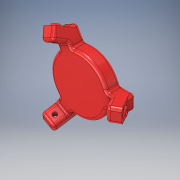
# Autodesk Inventor part: BottomPlatform
Saved by Autodesk Inventor 2019 (Build 230136000, 136)
## iProperties
Created: 2022-07-06
Part Number: BottomPlatform
Material: Generic
Document SubType Name: Modeling
Designer: zreik
Density: 1 g/cm^3
Appearance: Light Red
Author: zreik
Autodesk Inventor part; units mm, degrees
ref_plane "YZ Plane" through (0, 0, 0) normal (1, 0, 0) x (0, 1, 0)
ref_plane "XZ Plane" through (0, 0, 0) normal (0, 1, 0) x (-1, 0, 0)
ref_plane "XY Plane" through (0, 0, 0) normal (0, 0, 1) x (1, 0, 0)
sketch "Sketch1" plane through (0, 0, 0) normal (0, 0, 1) x (1, 0, 0)
  circle A0 centre (0, 0) radius 20
  line L0 (10, -5) -> (30, -5)
  line L1 (30, -5) -> (30, 5)
  line L2 (30, 5) -> (10, 5)
  line L3 (10, 5) -> (10, -5)
  line L4 (10, -5) -> (30, 5) construction
  line L5 (30, -5) -> (10, 5) construction
  point P0 (20, 0)
  dimension "d0" = 40
  dimension "d3" = 10
  dimension "d4" = 20
  dimension "d5" = 0
  constraints: 12 end point, 2 midpoint, 2 parallel, 1 coincident, 1 horizontal, 1 horizontal alignment, 1 perpendicular, 2 other
  measures "d3" distance of L0.end L1.end
  measures "d4" distance of L0.start L0.end
  measures "d5" vertical distance of point (0, 0) point (20, 0)
extrude "Extrusion1" add sketch "Sketch1" along normal mid plane 10 contours A0 L0 L3 L2 | L2 L3 L0 A0
extrude "Extrusion2" add sketch "Sketch1" along normal mid plane 10 contours A0 L0 L3 L2 | A0 L2 L1 L0 picked at (13.3333, 0)
chamfer "Chamfer1" distance 7 angle 30 1 edges at (30, 0, 5) measured on face at (6.3805, 10.8065, 5)
sketch "Sketch2" plane through (23, -5, 5) normal (0.5, 0, 0.8660254) x (0.8660254, 0, -0.5)
  line L0 (8.0829, 0) -> (0, 0)
  line L1 (0, 0) -> (0, 10)
  line L2 (0, 10) -> (8.0829, 10)
  line L3 (8.0829, 10) -> (8.0829, 0)
  line L4 (8.0829, 0) -> (0, 10) construction
  line L5 (0, 0) -> (8.0829, 10) construction
  line L6 (0, 10) -> (0, 0) projected
  line L7 (8.0829, 0) -> (8.0829, 10) projected
  line L8 (8.0829, 10) -> (0, 10) projected
  line L9 (0, 0) -> (8.0829, 0) projected
  point P0 (-17.4186, 5)
  point P1 (4.0415, 5)
  dimension "d11" = 0
  dimension "d12" = 0
  dimension "d13" = 0
  dimension "d14" = 0
  constraints: 12 end point, 2 midpoint, 2 parallel, 1 horizontal, 1 perpendicular
  measures "d11" distance between parallel lines of L1 L6
  measures "d12" distance between parallel lines of L7 L3
  measures "d13" distance between parallel lines of L8 L2
  measures "d14" distance between parallel lines of L9 L0
extrude "Extrusion3" add sketch "Sketch2" along normal blind 10
sketch "Sketch3" plane through (23, -5, 5) normal (-0.8660254, 0, 0.5) x (0.5, 0, 0.8660254)
  circle A0 centre (5, 5) radius 1.5
  line L0 (10, 10) -> (10, 0) projected
  line L1 (0, 10) -> (0, 0) projected
  line L2 (0, 0) -> (10, 0) projected
  line L3 (0, 10) -> (10, 10) projected
  point P0 (-15.8301, 5)
  dimension "d17" = 3
  dimension "d18" = 5
  dimension "d19" = 5
  dimension "d20" = 5
  dimension "d21" = 5
  constraints: 1 centre point
  measures "d17" diameter of A0
  measures "d18" distance from line of L0 A0.centre
  measures "d19" distance from line of L1 A0.centre
  measures "d20" distance from line of L2 A0.centre
  measures "d21" distance from line of L3 A0.centre
extrude "Extrusion8" cut sketch "Sketch3" against normal through all contours A0
sketch "Sketch6" plane through (30, -5, 0.9585) normal (0.8660254, 0, -0.5) x (-0.5, 0, -0.8660254)
  circle A0 centre (-5, 5) radius 3.5
  circle A1 centre (-5, 5) radius 1.5 projected
  point P0 (15.8301, 5)
  dimension "d40" = 7
  constraints: 1 centre point, 1 concentric
  measures "d40" diameter of A0
extrude "Extrusion9" add sketch "Sketch6" along normal blind 1.158
chamfer "Chamfer3" distance 1 angle 45 1 edges at (35.2529, 0, 7.7408)
pattern_circular "Circular Pattern1" count 3 over 360 about axis through (0, 0, 0) along (0, 0, 1) of "Extrusion3", "Extrusion2", "Chamfer1", "Extrusion8", "Chamfer3", "Extrusion9"
fillet "Fillet1" radius 2 9 edges at (30, 0, -5) (-15, 25.9808, -5) (-15, -25.9808, -5) (19.3649, 5, 0) (-5.3523, 19.2705, 0) (19.3649, -5, 0) (-5.3523, -19.2705, 0) (-14.0126, -14.2705, 0) (-14.0126, 14.2705, 0)
fillet "Fillet2" radius 2 3 edges at (-11.5, -19.9186, 5) (23, 0, 5) (-11.5, 19.9186, 5)
fillet "Fillet3" radius 2 3 edges at (-14, 24.2487, 13.6603) (28, 0, 13.6603) (-14, -24.2487, 13.6603)
fillet "Fillet4" radius 2 39 edges at (-18.4373, 21.9344, 12.8601) (-16.9745, 19.4006, 8.9641) (-15.7528, 17.2846, 5.2679) (-15.0056, 15.9905, 5) (-14.5005, 14.3629, 5) (-20, 0, 5) (-14.5005, -14.3629, 5) (-15.0056, -15.9905, 5) (-15.7528, -17.2846, 5.2679) (-16.9745, -19.4006, 8.9641) (-18.4373, -21.9344, 12.8601) (-20.5131, -25.5298, 11.1395) (-20.5131, 25.5298, 11.1395) (-11.8529, 30.5298, 11.1395) (-8.3142, 24.4006, 8.9641) (-7.0925, 22.2846, 5.2679) (-6.3454, 20.9905, 5) (-5.1884, 19.7392, 5) (10, 17.3205, 5) (19.6889, 5.3763, 5) (21.351, 5, 5) (22.8453, 5, 5.2679) (25.2887, 5, 8.9641) (28.2144, 5, 12.8601) (32.366, 5, 11.1395) (-9.7771, 26.9344, 12.8601) (28.2144, -5, 12.8601) (25.2887, -5, 8.9641) (22.8453, -5, 5.2679) (21.351, -5, 5) (19.6889, -5.3763, 5) (10, -17.3205, 5) (-5.1884, -19.7392, 5) (-6.3454, -20.9905, 5) (-7.0925, -22.2846, 5.2679) (-8.3142, -24.4006, 8.9641) (-9.7771, -26.9344, 12.8601) (-11.8529, -30.5298, 11.1395) (32.366, -5, 11.1395)
fillet "Fillet5" radius 2 27 edges at (-16.5443, -18.6556, -5) (-14.5005, -14.3629, -5) (-20, 0, -5) (-14.5005, 14.3629, -5) (-16.5443, 18.6556, -5) (-19.0372, 22.9735, -4.4142) (-19.3301, 23.4808, -1.0207) (-19.3301, -23.4808, -1.0207) (-19.0372, -22.9735, -4.4142) (-5.1884, -19.7392, -5) (-7.884, -23.6556, -5) (-10.377, -27.9735, -4.4142) (-10.6699, -28.4808, -1.0207) (19.6889, -5.3763, -5) (24.4283, -5, -5) (29.4142, -5, -4.4142) (30, -5, -1.0207) (10, -17.3205, -5) (19.6889, 5.3763, -5) (24.4283, 5, -5) (29.4142, 5, -4.4142) (30, 5, -1.0207) (-5.1884, 19.7392, -5) (-7.884, 23.6556, -5) (-10.377, 27.9735, -4.4142) (-10.6699, 28.4808, -1.0207) (10, 17.3205, -5)
equation "\"d18\" = d19"
equation "\"d20\" = d21"
body "Solid1"
